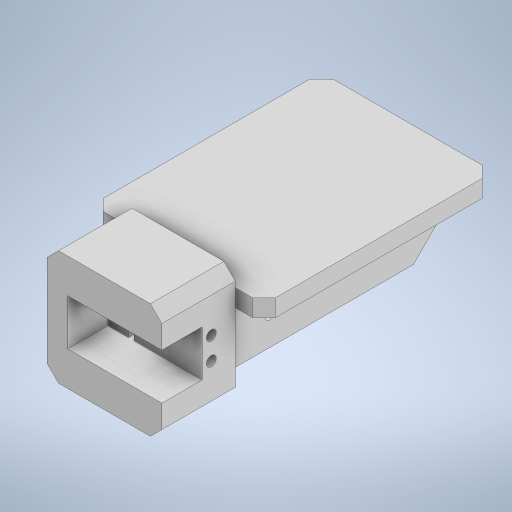
# Autodesk Inventor part: ES117_MP1
Saved by Autodesk Inventor 2024 (Build 280153000, 153)
## iProperties
Created: 2023-06-04
Part Number: ES117_MP1
Material: Generic
Document SubType Name: Modeling
Designer: vilas
Density: 1 g/cm^3
Appearance: Default
Author: vilas
Autodesk Inventor part; units mm, degrees
ref_plane "YZ Plane" through (0, 0, 0) normal (1, 0, 0) x (0, 1, 0)
ref_plane "XZ Plane" through (0, 0, 0) normal (0, 1, 0) x (-1, 0, 0)
ref_plane "XY Plane" through (0, 0, 0) normal (0, 0, 1) x (1, 0, 0)
sketch "Sketch1" plane through (0, 0, 0) normal (0, 0, 1) x (1, 0, 0)
  line L0 (0, 0) -> (50, 0)
  line L1 (50, 0) -> (50, 50)
  line L2 (50, 50) -> (0, 50)
  line L3 (0, 50) -> (0, 0)
  dimension "d0" = 50
  dimension "d1" = 50
  constraints: 8 end point, 2 parallel, 1 horizontal, 1 perpendicular
  measures "d0" distance of L2.end L1.end
  measures "d1" distance of L1.end L0.end
extrude "Extrusion1" add sketch "Sketch1" along normal blind 32
sketch "Sketch2" plane through (0, 0, 32) normal (0, 0, 1) x (1, 0, 0)
  line L0 (50, 0) -> (50, 50) projected
  line L1 (50, 15) -> (9, 15)
  line L2 (9, 15) -> (9, 35)
  line L3 (9, 35) -> (50, 35)
  line L4 (50, 35) -> (50, 15)
  line L5 (0, 0) -> (50, 0) projected
  point P0 (50, 35)
  dimension "d4" = 41
  dimension "d5" = 20
  dimension "d6" = 15
  constraints: 8 end point, 2 parallel, 1 horizontal, 1 perpendicular, 1 point on line
  measures "d4" distance of L2.end L3.end
  measures "d5" distance of L1.end L2.end
  measures "d6" distance between parallel lines of L5 L1
extrude "Extrusion2" cut sketch "Sketch2" against normal blind 17.5
sketch "Sketch3" plane through (0, 0, 0) normal (-1, 0, 0) x (0, 0, 1)
  line L0 (32, 50) -> (32, 0) projected
  line L1 (32, 35) -> (10.5, 35) construction
  line L2 (32, 35) -> (53.5, 35) construction
  line L3 (10.5, 35) -> (10.5, 15) construction
  line L4 (10.5, 15) -> (32, 15) construction
  line L5 (0, 50) -> (32, 50) projected
  line L6 (32, 29.85) -> (10.5, 29.85) construction
  line L7 (32, 20.15) -> (10.5, 20.15) construction
  point P0 (0, 0)
  dimension "d9" = 21.5
  dimension "d10" = 180
  dimension "d11" = 20
  dimension "d12" = 15
  dimension "d13" = 5.15
  dimension "d14" = 5.15
  constraints: 12 end point, 6 point on line, 3 horizontal, 3 perpendicular, 1 collinear
  measures "d9" distance of L1.start L1.end
  measures "d10" angle of L1 L2
  measures "d11" distance of L1.end L3.end
  measures "d12" distance between parallel lines of L5 L1
  measures "d13" distance between parallel lines of L6 L1
  measures "d14" distance between parallel lines of L4 L7
hole "Hole1" at (0, 29.85, 10.5) at (0, 20.15, 10.5) direction (1, 0, 0) diameter 4.3 end through all
sketch "Sketch4" plane through (0, 0, 14.5) normal (0, 0, 1) x (1, 0, 0)
  line L0 (9, 35) -> (50, 35) projected
  line L1 (50, 15) -> (9, 15) projected
  line L2 (18, 35) -> (20.4, 35)
  line L3 (20.4, 35) -> (20.4, 15)
  line L4 (20.4, 15) -> (18, 15)
  line L5 (18, 15) -> (18, 35)
  line L6 (9, 15) -> (9, 35) projected
  point P0 (0, 0)
  point P1 (18, 15)
  dimension "d22" = 9
  dimension "d23" = 2.4
  constraints: 8 end point, 2 parallel, 2 point on line, 1 horizontal, 1 perpendicular
  measures "d22" distance between parallel lines of L5 L6
  measures "d23" distance between parallel lines of L3 L5
extrude "Extrusion3" cut sketch "Sketch4" against normal blind 7 contours L0 L3 L1 L5
chamfer "Chamfer1" distance 5 angle 45 4 edges at (0, 50, 16) (50, 50, 16) (0, 0, 16) (50, 0, 16)
sketch "Sketch7" plane through (0, 0, 14.5) normal (0, 0, 1) x (1, 0, 0)
  line L0 (18, 15) -> (18, 35) projected
  line L1 (18, 24.5) -> (16, 24.5)
  line L2 (16, 24.5) -> (16, 25.5)
  line L3 (16, 25.5) -> (18, 25.5)
  line L4 (18, 25.5) -> (18, 24.5)
  line L5 (9, 35) -> (50, 35) projected
  point P0 (0, 0)
  dimension "d45" = 2
  dimension "d46" = 1
  dimension "d47" = 9.5
  constraints: 8 end point, 2 parallel, 1 horizontal, 1 perpendicular, 1 point on line
  measures "d45" distance of L2.end L3.end
  measures "d46" distance of L1.end L2.end
  measures "d47" distance between parallel lines of L3 L5
extrude "Extrusion5" cut sketch "Sketch7" against normal blind 7
chamfer "Chamfer3" distance 7 distance2 2 1 edges at (16, 25, 7.5) measured on face at (16, 25.1667, 12.1667)
sketch "Sketch9" plane through (0, 0, 0) normal (0, 0, -1) x (-1, 0, 0)
  line L0 (-45, 50) -> (-5, 50) projected
  line L1 (-25, 50) -> (-25, 0) construction
  line L2 (-5, 0) -> (-45, 0) projected
  line L3 (-37.5, 0) -> (-37.5, 42.5)
  line L4 (-37.5, 42.5) -> (-12.5, 42.5)
  line L5 (-12.5, 42.5) -> (-12.5, 0)
  point P0 (0, 0)
  dimension "d61" = 42.5
  dimension "d62" = 25
  dimension "d63" = 12.5
  constraints: 8 end point, 2 midpoint, 2 perpendicular, 2 point on line, 1 vertical
  measures "d61" distance of L3.start L3.end
  measures "d62" distance of L3.end L4.end
  measures "d63" distance between parallel lines of L1 L3
extrude "Extrusion6" add sketch "Sketch9" along normal blind 100
sketch "Sketch10" plane through (12.5, 0, 0) normal (-1, 0, 0) x (0, 0, 1)
  line L0 (-100, 42.5) -> (-100, 0) projected
  line L1 (-100, 42.5) -> (0, 42.5)
  line L2 (0, 42.5) -> (0, 35)
  line L3 (0, 35) -> (-100, 35)
  line L4 (-100, 35) -> (-100, 42.5)
  point P0 (0, 0)
  dimension "d66" = 100
  dimension "d67" = 7.5
  constraints: 8 end point, 2 parallel, 1 horizontal, 1 perpendicular
  measures "d66" distance of L2.end L3.end
  measures "d67" distance of L1.end L2.end
extrude "Extrusion7" add sketch "Sketch10" along normal blind 25 and the other way blind 50
chamfer "Chamfer4" distance 5 angle 45 4 edges at (-12.5, 38.75, 0) (-12.5, 38.75, -100) (62.5, 38.75, 0) (62.5, 38.75, -100)
chamfer "Chamfer5" distance 10 angle 45 1 edges at (25, 0, -100)
sketch "Sketch11" plane through (12.5, 0, 0) normal (-1, 0, 0) x (0, 0, 1)
  line L0 (-100, 10) -> (-100, 35) projected
  line L1 (-100, 12.5) -> (0, 12.5) construction
  line L2 (0, 0) -> (-90, 0) projected
  line L3 (-27.5, 0) -> (-27.5, 35) construction
  line L4 (-90, 0) -> (-90, 35) construction
  line L5 (-95, 35) -> (-5, 35) projected
  line L6 (0, 35) -> (0, 5) projected
  circle A0 centre (-90, 12.5) radius 2.15
  circle A1 centre (-27.5, 12.5) radius 2.15
  dimension "d78" = 12.5
  dimension "d79" = 27.5
  dimension "d80" = 10
  dimension "d81" = 4.3
  dimension "d82" = 4.3
  constraints: 8 point on line, 6 end point, 2 centre point, 2 vertical, 1 horizontal
  measures "d78" distance between parallel lines of L2 L1
  measures "d79" distance between parallel lines of L3 L6
  measures "d80" distance between parallel lines of L4 L0
  measures "d81" diameter of A0
  measures "d82" diameter of A1
extrude "Extrusion8" cut sketch "Sketch11" against normal through all
body "Solid1"
